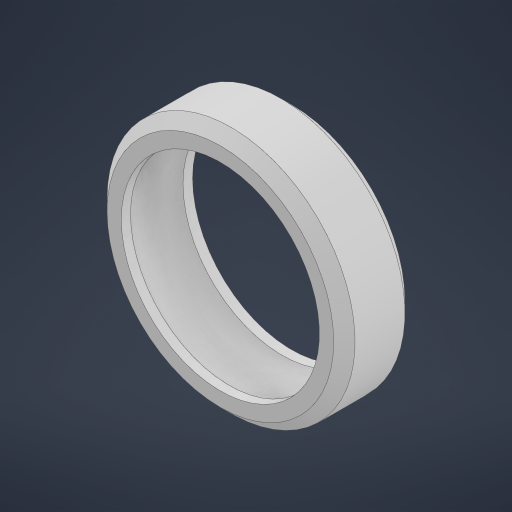
# Autodesk Inventor part: 5mm Bearing Outside
Saved by Autodesk Inventor 2023 (Build 270158000, 158)
## iProperties
Created: 2022-10-15
Part Number: 5mm Bearing Outside
Material: Generic
Document SubType Name: Modeling
Designer: izack
Density: 1 g/cm^3
Appearance: Default
Author: izack
## iProperties of the stored document 5mm Bearing Outside_3DPrint.ipt
Part Number: 5mm Bearing Outside_3DPrint
Material: Generic
Document SubType Name: Modeling
Designer: izack
Appearance: Default
Author: izack
Autodesk Inventor part; units mm, degrees
ref_plane "YZ Plane" through (0, 0, 0) normal (1, 0, 0) x (0, 1, 0)
ref_plane "XZ Plane" through (0, 0, 0) normal (0, 1, 0) x (-1, 0, 0)
ref_plane "XY Plane" through (0, 0, 0) normal (0, 0, 1) x (1, 0, 0)
sketch "Sketch1" plane through (0, 0, 0) normal (0, 1, 0) x (-1, 0, 0)
  line L0 (-3.2, 2.5) -> (3.2, 2.5)
  line L1 (3.2, -2.5) -> (-3.2, -2.5)
  line L2 (-3.2, -2.5) -> (-3.2, 2.5)
  line L3 (-3.2, 2.5) -> (3.2, -2.5) construction
  line L4 (3.2, 2.5) -> (-3.2, -2.5) construction
  circle A0 centre (5.45, 0.0144) radius 2.375
  line L5 (7.7, 2.5) -> (7.7, -2.5)
  line L6 (7.7, -2.5) -> (6.95, -2.5)
  line L7 (6.95, -2.5) -> (6.95, -1.8269)
  line L8 (7.7, 2.5) -> (6.95, 2.5)
  line L9 (6.95, 2.5) -> (6.95, 1.8558)
  line L10 (7.7, 2.5) -> (8.7, 2.5)
  line L11 (8.7, 2.5) -> (8.7, -2.5)
  line L12 (8.7, -2.5) -> (7.7, -2.5)
  line L13 (7.7, -2.5) -> (7.7, 2.5)
  line L14 (0, 2.5) -> (0, -2.5)
  line L15 (3.2, -2.5) -> (3.2, 2.5)
  point P0 (0, 0)
  dimension "d1" = 6.4
  dimension "d2" = 5
  dimension "d3" = 4.75
  dimension "d4" = 2.25
  dimension "d5" = 0.75
  dimension "d6" = 1
  dimension "d11" = 2.25
  constraints: 32 end point, 4 midpoint, 3 horizontal, 3 parallel, 3 perpendicular, 2 point on circle, 2 point on line, 2 vertical, 1 centre point
  measures "d1" distance of L1.start L1.end
  measures "d2" distance of L0.end L1.start
  measures "d3" diameter of A0
  measures "d4" distance from line of A0.centre L5
  measures "d5" distance of L5.end L6.end
  measures "d6" distance of L11.end L12.end
  measures "d11" distance from line of L15 A0.centre
revolve "Revolution1" add sketch "Sketch1" angle 360 about axis through (0, 0, 2.5) along (0, 0, -1) contours L9 L8 L5 A0 | L5 L10 L11 L12 A0 | A0 L5 L6 L7
chamfer "Chamfer1" distance 0.75 angle 45 2 edges at (8.7, 0, -2.5) (8.7, 0, 2.5)
body "Solid1"
